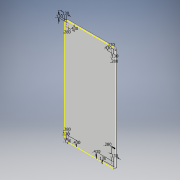
# Autodesk Inventor part: InnerDoorCover
Saved by Autodesk Inventor 2019 (Build 230136000, 136)
## iProperties
Created: 2019-02-25
Part Number: InnerDoorCover
Material: Generic
Document SubType Name: Modeling
Designer: garretthagen21
Density: 1 g/cm^3
Appearance: Default
Author: garretthagen21
Autodesk Inventor part; units mm, degrees
ref_plane "YZ Plane" through (0, 0, 0) normal (1, 0, 0) x (0, 1, 0)
ref_plane "XZ Plane" through (0, 0, 0) normal (0, 1, 0) x (-1, 0, 0)
ref_plane "XY Plane" through (0, 0, 0) normal (0, 0, 1) x (1, 0, 0)
sketch "Base" plane through (0, 0, 0) normal (0, 0, 1) x (1, 0, 0)
  line L0 (-5.5432, 7.38) -> (85.3888, 7.38)
  line L1 (88.5638, 4.205) -> (88.5638, -189.343)
  line L2 (85.3888, -192.518) -> (-5.5432, -192.518)
  line L3 (-8.7182, -189.343) -> (-8.7182, 4.205)
  arc A0 (-5.5432, 7.38) -> (-8.7182, 4.205) centre (-5.5432, 4.205) ccw
  arc A1 (88.5638, 4.205) -> (85.3888, 7.38) centre (85.3888, 4.205) ccw
  arc A2 (85.3888, -192.518) -> (88.5638, -189.343) centre (85.3888, -189.343) ccw
  arc A3 (-8.7182, -189.343) -> (-5.5432, -192.518) centre (-5.5432, -189.343) ccw
  point P0 (0, 0)
  point P1 (88.5638, -192.518)
  point P2 (88.5638, 7.38)
  point P3 (-8.7182, -192.518)
  dimension "d0" = 97.282
  dimension "d1" = 199.898
  dimension "d2" = 3.175
  constraints: 8 end point, 8 point on circle, 8 tangent, 6 point on line, 4 centre point, 3 equal radius, 2 parallel, 1 horizontal, 1 perpendicular
  measures "d0" distance of point (88.564, -192.518) point (-8.718, -192.518)
  measures "d1" distance of point (88.564, 7.38) point (88.564, -192.518)
  measures "d2" radius of A0
extrude "Extrusion1" add sketch "Base" along normal blind 2.54
sketch "Sketch2" plane through (0, 0, 2.54) normal (0, 0, 1) x (1, 0, 0)
  line L0 (85.3888, 7.38) -> (-5.5432, 7.38) projected
  line L1 (-8.7182, 4.205) -> (-8.7182, -189.343) projected
  line L2 (88.5638, -189.343) -> (88.5638, 4.205) projected
  line L3 (-5.5432, -192.518) -> (85.3888, -192.518) projected
  point P0 (0, 0)
  point P1 (-5.4162, 4.078)
  point P2 (85.2618, 4.078)
  point P3 (-5.4162, -189.216)
  point P4 (85.2618, -189.216)
  point P5 (-1.6062, -3.542)
  point P6 (81.4518, -3.542)
  point P7 (81.4518, -181.596)
  point P8 (-1.6062, -181.596)
  dimension "d5" = 3.302
  dimension "d6" = 3.302
  dimension "d7" = 3.302
  dimension "d8" = 3.302
  dimension "d9" = 3.302
  dimension "d10" = 3.302
  dimension "d11" = 3.302
  dimension "d12" = 3.302
  dimension "d13" = 10.922
  dimension "d14" = 7.112
  dimension "d15" = 7.112
  dimension "d16" = 10.922
  dimension "d17" = 10.922
  dimension "d18" = 7.112
  dimension "d19" = 10.922
  dimension "d20" = 7.112
  measures "d5" distance from line of L0 point (-5.416, 4.078)
  measures "d6" distance from line of L1 point (-5.416, 4.078)
  measures "d7" distance from line of point (85.262, 4.078) L0
  measures "d8" distance from line of point (85.262, 4.078) L2
  measures "d9" distance from line of L3 point (85.262, -189.216)
  measures "d10" distance from line of point (85.262, -189.216) L2
  measures "d11" distance from line of L1 point (-5.416, -189.216)
  measures "d12" distance from line of L3 point (-5.416, -189.216)
  measures "d13" distance from line of L0 point (-1.606, -3.542)
  measures "d14" distance from line of L1 point (-1.606, -3.542)
  measures "d15" distance from line of L2 point (81.452, -3.542)
  measures "d16" distance from line of L0 point (81.452, -3.542)
  measures "d17" distance from line of L3 point (81.452, -181.596)
  measures "d18" distance from line of L2 point (81.452, -181.596)
  measures "d19" distance from line of L3 point (-1.606, -181.596)
  measures "d20" distance from line of L1 point (-1.606, -181.596)
body "Solid1"
